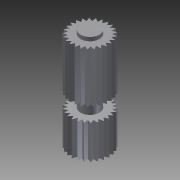
# Autodesk Inventor part: launcher.motor.midgear
Saved by Autodesk Inventor 2011 (Build 150239000, 239)
## iProperties
Created: 2011-04-05
Part Number: launcher.motor.midgear
Document SubType Name: Modeling
Designer: Rob
Density: 1 g/cm^3
Author: Rob
Autodesk Inventor part; units mm, degrees
ref_plane "YZ Plane" through (0, 0, 0) normal (1, 0, 0) x (0, 1, 0)
sketch "Sketch1" plane through (0, 0, 0) normal (0, 0, 1) x (1, 0, 0)
  circle A0 centre (0, 0) radius 0.75
  dimension "d0" = 1.5
  constraints: 1 centre point, 1 coincident
  measures "d0" diameter of A0
extrude "Extrusion1" add sketch "Sketch1" along normal blind 8.4
ref_plane "Work Plane1" through (0, 0, 8.1) normal (0, 0, 1) x (1, 0, 0)
sketch "Sketch2" plane through (0, 0, 8.1) normal (0, 0, 1) x (1, 0, 0)
  circle A0 centre (0, 0) radius 1.25
  dimension "d10" = 2.5
  constraints: 1 centre point, 1 coincident
  measures "d10" diameter of A0
extrude "Extrusion2" add sketch "Sketch2" against normal blind 4
ref_plane "Work Plane2" through (0, 0, 0.3) normal (0, 0, -1) x (-1, 0, 0)
sketch "Sketch3" plane through (0, 0, 0.3) normal (0, 0, -1) x (-1, 0, 0)
  circle A0 centre (0, 0) radius 1.25
  dimension "d7" = 2.5
  constraints: 1 centre point, 1 coincident
  measures "d7" diameter of A0
extrude "Extrusion3" add sketch "Sketch3" against normal blind 2.7
sketch "Sketch4" plane through (0, 0, 0.3) normal (0, 0, -1) x (-1, 0, 0)
  circle A0 centre (0, 0) radius 1.25 projected
  circle A1 centre (0, 0) radius 0.75 projected
  line L0 (0, 0) -> (-2.2024, 0)
  line L1 (-1.5572, 0) -> (-1.2398, -0.1597)
  line L2 (-1.5572, 0) -> (-1.2398, 0.1597)
  arc A2 (-1.2398, 0.1597) -> (-1.2398, -0.1597) centre (0, 0) ccw
  line L3 (-1.2398, -0.1597) -> (-1.5572, 0)
  line L4 (-1.2398, 0.1597) -> (-1.5572, 0)
  arc A3 (-1.2405, -0.1536) -> (-1.1611, -0.463) centre (0, 0) ccw
  line L5 (-1.1611, -0.463) -> (-1.5083, -0.3873)
  line L6 (-1.2405, -0.1536) -> (-1.5083, -0.3873)
  arc A4 (-1.1634, -0.4573) -> (-1.0095, -0.7372) centre (0, 0) ccw
  line L7 (-1.0095, -0.7372) -> (-1.3646, -0.7502)
  line L8 (-1.1634, -0.4573) -> (-1.3646, -0.7502)
  arc A5 (-1.0131, -0.7322) -> (-0.7944, -0.9651) centre (0, 0) ccw
  line L9 (-0.7944, -0.9651) -> (-1.1351, -1.066)
  line L10 (-1.0131, -0.7322) -> (-1.1351, -1.066)
  arc A6 (-0.7992, -0.9612) -> (-0.5294, -1.1323) centre (0, 0) ccw
  line L11 (-0.5294, -1.1323) -> (-0.8344, -1.3148)
  line L12 (-0.7992, -0.9612) -> (-0.8344, -1.3148)
  arc A7 (-0.535, -1.1297) -> (-0.2312, -1.2284) centre (0, 0) ccw
  line L13 (-0.2312, -1.2284) -> (-0.4812, -1.481)
  line L14 (-0.535, -1.1297) -> (-0.4812, -1.481)
  arc A8 (-0.2373, -1.2273) -> (0.0816, -1.2473) centre (0, 0) ccw
  line L15 (0.0816, -1.2473) -> (-0.0978, -1.5541)
  line L16 (-0.2373, -1.2273) -> (-0.0978, -1.5541)
  arc A9 (0.0754, -1.2477) -> (0.3892, -1.1879) centre (0, 0) ccw
  line L17 (0.3892, -1.1879) -> (0.2918, -1.5296)
  line L18 (0.0754, -1.2477) -> (0.2918, -1.5296)
  arc A10 (0.3833, -1.1898) -> (0.6724, -1.0538) centre (0, 0) ccw
  line L19 (0.6724, -1.0538) -> (0.663, -1.409)
  line L20 (0.3833, -1.1898) -> (0.663, -1.409)
  arc A11 (0.6672, -1.0571) -> (0.9133, -0.8534) centre (0, 0) ccw
  line L21 (0.9133, -0.8534) -> (0.9926, -1.1998)
  line L22 (0.6672, -1.0571) -> (0.9926, -1.1998)
  arc A12 (0.9091, -0.8579) -> (1.0969, -0.5995) centre (0, 0) ccw
  line L23 (1.0969, -0.5995) -> (1.2598, -0.9153)
  line L24 (0.9091, -0.8579) -> (1.2598, -0.9153)
  arc A13 (1.0939, -0.6049) -> (1.2115, -0.3079) centre (0, 0) ccw
  line L25 (1.2115, -0.3079) -> (1.4478, -0.5732)
  line L26 (1.0939, -0.6049) -> (1.4478, -0.5732)
  arc A14 (1.21, -0.3139) -> (1.25, 0.0031) centre (0, 0) ccw
  line L27 (1.25, 0.0031) -> (1.5449, -0.1952)
  line L28 (1.21, -0.3139) -> (1.5449, -0.1952)
  arc A15 (1.25, -0.0031) -> (1.21, 0.3139) centre (0, 0) ccw
  line L29 (1.21, 0.3139) -> (1.5449, 0.1952)
  line L30 (1.25, -0.0031) -> (1.5449, 0.1952)
  arc A16 (1.2115, 0.3079) -> (1.0939, 0.6049) centre (0, 0) ccw
  line L31 (1.0939, 0.6049) -> (1.4478, 0.5732)
  line L32 (1.2115, 0.3079) -> (1.4478, 0.5732)
  arc A17 (1.0969, 0.5995) -> (0.9091, 0.8579) centre (0, 0) ccw
  line L33 (0.9091, 0.8579) -> (1.2598, 0.9153)
  line L34 (1.0969, 0.5995) -> (1.2598, 0.9153)
  arc A18 (0.9133, 0.8534) -> (0.6672, 1.0571) centre (0, 0) ccw
  line L35 (0.6672, 1.0571) -> (0.9926, 1.1998)
  line L36 (0.9133, 0.8534) -> (0.9926, 1.1998)
  arc A19 (0.6724, 1.0538) -> (0.3833, 1.1898) centre (0, 0) ccw
  line L37 (0.3833, 1.1898) -> (0.663, 1.409)
  line L38 (0.6724, 1.0538) -> (0.663, 1.409)
  arc A20 (0.3892, 1.1879) -> (0.0754, 1.2477) centre (0, 0) ccw
  line L39 (0.0754, 1.2477) -> (0.2918, 1.5296)
  line L40 (0.3892, 1.1879) -> (0.2918, 1.5296)
  arc A21 (0.0816, 1.2473) -> (-0.2373, 1.2273) centre (0, 0) ccw
  line L41 (-0.2373, 1.2273) -> (-0.0978, 1.5541)
  line L42 (0.0816, 1.2473) -> (-0.0978, 1.5541)
  arc A22 (-0.2312, 1.2284) -> (-0.535, 1.1297) centre (0, 0) ccw
  line L43 (-0.535, 1.1297) -> (-0.4812, 1.481)
  line L44 (-0.2312, 1.2284) -> (-0.4812, 1.481)
  arc A23 (-0.5294, 1.1323) -> (-0.7992, 0.9612) centre (0, 0) ccw
  line L45 (-0.7992, 0.9612) -> (-0.8344, 1.3148)
  line L46 (-0.5294, 1.1323) -> (-0.8344, 1.3148)
  arc A24 (-0.7944, 0.9651) -> (-1.0131, 0.7322) centre (0, 0) ccw
  line L47 (-1.0131, 0.7322) -> (-1.1351, 1.066)
  line L48 (-0.7944, 0.9651) -> (-1.1351, 1.066)
  arc A25 (-1.0095, 0.7372) -> (-1.1634, 0.4573) centre (0, 0) ccw
  line L49 (-1.1634, 0.4573) -> (-1.3646, 0.7502)
  line L50 (-1.0095, 0.7372) -> (-1.3646, 0.7502)
  arc A26 (-1.1611, 0.463) -> (-1.2405, 0.1536) centre (0, 0) ccw
  line L51 (-1.2405, 0.1536) -> (-1.5083, 0.3873)
  line L52 (-1.1611, 0.463) -> (-1.5083, 0.3873)
  dimension "d13" = 360
  constraints: 106 end point, 50 point on circle, 25 centre point, 2 coincident, 2 collinear, 1 horizontal, 1 point on line, 1 symmetric about line, 176 other
extrude "Extrusion4" add sketch "Sketch4" against normal up to surface (2.7 mm away) contours A0 L27 L30 | A0 L32 L29 L30 L27 | L30 L27 L28 L25 A0 | A0 L29 L32 | L25 L28 A0 | A0 L34 L31 L32 L29 | L28 L25 L26 L23 A0 | A0 L31 L34 | L23 L26 A0 | A0 L36 L33 L34 L31 | L26 L23 L24 L21 A0 | A0 L33 L36 | L21 L24 A0 | A0 L38 L35 L36 L33 | L24 L21 L22 L19 A0 | A0 L35 L38 | L19 L22 A0 | A0 L40 L37 L38 L35 | L22 L19 L20 L17 A0 | A0 L37 L40 | L17 L20 A0 | A0 L42 L39 L40 L37 | L20 L17 L18 L15 A0 | A0 L39 L42 | L15 L18 A0 | A0 L44 L41 L42 L39 | L18 L15 L16 L13 A0 | A0 L41 L44 | L13 L16 A0 | A0 L46 L43 L44 L41 | L16 L13 L14 L11 A0 | A0 L43 L46 | L11 L14 A0 | A0 L48 L45 L46 L43 | L14 L11 L12 L9 A0 | A0 L45 L48 | L9 L12 A0 | A0 L50 L47 L48 L45 | L12 L9 L10 L7 A0 | A0 L47 L50 | L7 L10 A0 | A0 L52 L49 L50 L47 | L10 L7 L8 L5 A0 | A0 L49 L52 | L5 L8 A0 | A0 L2 L51 L52 L49 | L8 L5 L6 L1 A0 | A0 L51 L2 | L1 L6 A0 | A0 L0 L2 L51 | L6 L1 L0 A0
sketch "Sketch5" plane through (0, 0, 8.1) normal (0, 0, 1) x (1, 0, 0)
  circle A0 centre (0, 0) radius 1.25
  circle A1 centre (0, 0) radius 0.75
  line L0 (0, 0) -> (-2.2024, 0)
  line L1 (-1.5572, 0) -> (-1.2398, -0.1597)
  line L2 (-1.5572, 0) -> (-1.2398, 0.1597)
  arc A2 (-1.2398, 0.1597) -> (-1.2398, -0.1597) centre (0, 0) ccw
  line L3 (-1.2398, -0.1597) -> (-1.5572, 0)
  line L4 (-1.2398, 0.1597) -> (-1.5572, 0)
  line L5 (-1.1611, -0.463) -> (-1.5083, -0.3873)
  line L6 (-1.2405, -0.1536) -> (-1.5083, -0.3873)
  arc A3 (-1.2405, -0.1536) -> (-1.1611, -0.463) centre (0, 0) ccw
  line L7 (-1.0095, -0.7372) -> (-1.3646, -0.7502)
  line L8 (-1.1634, -0.4573) -> (-1.3646, -0.7502)
  arc A4 (-1.1634, -0.4573) -> (-1.0095, -0.7372) centre (0, 0) ccw
  line L9 (-0.7944, -0.9651) -> (-1.1351, -1.066)
  line L10 (-1.0131, -0.7322) -> (-1.1351, -1.066)
  arc A5 (-1.0131, -0.7322) -> (-0.7944, -0.9651) centre (0, 0) ccw
  line L11 (-0.5294, -1.1323) -> (-0.8344, -1.3148)
  line L12 (-0.7992, -0.9612) -> (-0.8344, -1.3148)
  arc A6 (-0.7992, -0.9612) -> (-0.5294, -1.1323) centre (0, 0) ccw
  line L13 (-0.2312, -1.2284) -> (-0.4812, -1.481)
  line L14 (-0.535, -1.1297) -> (-0.4812, -1.481)
  arc A7 (-0.535, -1.1297) -> (-0.2312, -1.2284) centre (0, 0) ccw
  line L15 (0.0816, -1.2473) -> (-0.0978, -1.5541)
  line L16 (-0.2373, -1.2273) -> (-0.0978, -1.5541)
  arc A8 (-0.2373, -1.2273) -> (0.0816, -1.2473) centre (0, 0) ccw
  line L17 (0.3892, -1.1879) -> (0.2918, -1.5296)
  line L18 (0.0754, -1.2477) -> (0.2918, -1.5296)
  arc A9 (0.0754, -1.2477) -> (0.3892, -1.1879) centre (0, 0) ccw
  line L19 (0.6724, -1.0538) -> (0.663, -1.409)
  line L20 (0.3833, -1.1898) -> (0.663, -1.409)
  arc A10 (0.3833, -1.1898) -> (0.6724, -1.0538) centre (0, 0) ccw
  line L21 (0.9133, -0.8534) -> (0.9926, -1.1998)
  line L22 (0.6672, -1.0571) -> (0.9926, -1.1998)
  arc A11 (0.6672, -1.0571) -> (0.9133, -0.8534) centre (0, 0) ccw
  line L23 (1.0969, -0.5995) -> (1.2598, -0.9153)
  line L24 (0.9091, -0.8579) -> (1.2598, -0.9153)
  arc A12 (0.9091, -0.8579) -> (1.0969, -0.5995) centre (0, 0) ccw
  line L25 (1.2115, -0.3079) -> (1.4478, -0.5732)
  line L26 (1.0939, -0.6049) -> (1.4478, -0.5732)
  arc A13 (1.0939, -0.6049) -> (1.2115, -0.3079) centre (0, 0) ccw
  line L27 (1.25, 0.0031) -> (1.5449, -0.1952)
  line L28 (1.21, -0.3139) -> (1.5449, -0.1952)
  arc A14 (1.21, -0.3139) -> (1.25, 0.0031) centre (0, 0) ccw
  line L29 (1.21, 0.3139) -> (1.5449, 0.1952)
  line L30 (1.25, -0.0031) -> (1.5449, 0.1952)
  arc A15 (1.25, -0.0031) -> (1.21, 0.3139) centre (0, 0) ccw
  line L31 (1.0939, 0.6049) -> (1.4478, 0.5732)
  line L32 (1.2115, 0.3079) -> (1.4478, 0.5732)
  arc A16 (1.2115, 0.3079) -> (1.0939, 0.6049) centre (0, 0) ccw
  line L33 (0.9091, 0.8579) -> (1.2598, 0.9153)
  line L34 (1.0969, 0.5995) -> (1.2598, 0.9153)
  arc A17 (1.0969, 0.5995) -> (0.9091, 0.8579) centre (0, 0) ccw
  line L35 (0.6672, 1.0571) -> (0.9926, 1.1998)
  line L36 (0.9133, 0.8534) -> (0.9926, 1.1998)
  arc A18 (0.9133, 0.8534) -> (0.6672, 1.0571) centre (0, 0) ccw
  line L37 (0.3833, 1.1898) -> (0.663, 1.409)
  line L38 (0.6724, 1.0538) -> (0.663, 1.409)
  arc A19 (0.6724, 1.0538) -> (0.3833, 1.1898) centre (0, 0) ccw
  line L39 (0.0754, 1.2477) -> (0.2918, 1.5296)
  line L40 (0.3892, 1.1879) -> (0.2918, 1.5296)
  arc A20 (0.3892, 1.1879) -> (0.0754, 1.2477) centre (0, 0) ccw
  line L41 (-0.2373, 1.2273) -> (-0.0978, 1.5541)
  line L42 (0.0816, 1.2473) -> (-0.0978, 1.5541)
  arc A21 (0.0816, 1.2473) -> (-0.2373, 1.2273) centre (0, 0) ccw
  line L43 (-0.535, 1.1297) -> (-0.4812, 1.481)
  line L44 (-0.2312, 1.2284) -> (-0.4812, 1.481)
  arc A22 (-0.2312, 1.2284) -> (-0.535, 1.1297) centre (0, 0) ccw
  line L45 (-0.7992, 0.9612) -> (-0.8344, 1.3148)
  line L46 (-0.5294, 1.1323) -> (-0.8344, 1.3148)
  arc A23 (-0.5294, 1.1323) -> (-0.7992, 0.9612) centre (0, 0) ccw
  line L47 (-1.0131, 0.7322) -> (-1.1351, 1.066)
  line L48 (-0.7944, 0.9651) -> (-1.1351, 1.066)
  arc A24 (-0.7944, 0.9651) -> (-1.0131, 0.7322) centre (0, 0) ccw
  line L49 (-1.1634, 0.4573) -> (-1.3646, 0.7502)
  line L50 (-1.0095, 0.7372) -> (-1.3646, 0.7502)
  arc A25 (-1.0095, 0.7372) -> (-1.1634, 0.4573) centre (0, 0) ccw
  line L51 (-1.2405, 0.1536) -> (-1.5083, 0.3873)
  line L52 (-1.1611, 0.463) -> (-1.5083, 0.3873)
  arc A26 (-1.1611, 0.463) -> (-1.2405, 0.1536) centre (0, 0) ccw
  dimension "d19" = 360
  constraints: 106 end point, 50 point on circle, 26 centre point, 2 coincident, 2 collinear, 1 horizontal, 1 point on line, 1 symmetric about line, 177 other
extrude "Extrusion5" add sketch "Sketch5" against normal up to surface (4 mm away) contours A0 L27 L30 | A0 L32 L29 L30 L27 | L30 L27 L28 L25 A0 | A0 L29 L32 | L25 L28 A0 | A0 L34 L31 L32 L29 | L28 L25 L26 L23 A0 | A0 L31 L34 | L23 L26 A0 | A0 L36 L33 L34 L31 | L26 L23 L24 L21 A0 | A0 L33 L36 | L21 L24 A0 | A0 L38 L35 L36 L33 | L24 L21 L22 L19 A0 | A0 L35 L38 | L19 L22 A0 | A0 L40 L37 L38 L35 | L22 L19 L20 L17 A0 | A0 L37 L40 | L17 L20 A0 | A0 L42 L39 L40 L37 | L20 L17 L18 L15 A0 | A0 L39 L42 | L15 L18 A0 | A0 L44 L41 L42 L39 | L18 L15 L16 L13 A0 | A0 L41 L44 | L13 L16 A0 | A0 L46 L43 L44 L41 | L16 L13 L14 L11 A0 | A0 L43 L46 | L11 L14 A0 | A0 L48 L45 L46 L43 | L14 L11 L12 L9 A0 | A0 L45 L48 | L9 L12 A0 | A0 L50 L47 L48 L45 | L12 L9 L10 L7 A0 | A0 L47 L50 | L7 L10 A0 | A0 L52 L49 L50 L47 | L10 L7 L8 L5 A0 | A0 L49 L52 | L5 L8 A0 | A0 L2 L51 L52 L49 | L8 L5 L6 L1 A0 | A0 L51 L2 | L1 L6 A0 | A0 L0 L2 L51 | L6 L1 L0 A0
body "Solid1"
